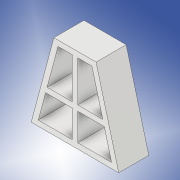
# Autodesk Inventor part: CA001
Saved by Autodesk Inventor 2017 (Build 210142000, 142)
## iProperties
Created: 2017-06-04
Part Number: CA001
Material: ABS Plastic
Document SubType Name: Modeling
Designer: Zach
Density: 1.06 g/cm^3
Appearance: CR White
Author: Zach
Autodesk Inventor part; units mm, degrees
ref_plane "YZ Plane" through (0, 0, 0) normal (1, 0, 0) x (0, 1, 0)
ref_plane "XZ Plane" through (0, 0, 0) normal (0, 1, 0) x (-1, 0, 0)
ref_plane "XY Plane" through (0, 0, 0) normal (0, 0, 1) x (1, 0, 0)
sketch "Sketch1" plane through (0, 0, 0) normal (0, 0, 1) x (1, 0, 0)
  line L0 (0, 0) -> (160, 0)
  line L1 (160, 0) -> (118.589, 154.5481)
  line L2 (41.411, 154.5481) -> (0, 0)
  line L3 (41.411, 154.5481) -> (118.589, 154.5481)
  dimension "d0" = 160
  dimension "d1" = 160
  dimension "d2" = 75
  dimension "d8" = 75
  constraints: 8 end point, 2 horizontal
  measures "d0" distance of L0.start L0.end
  measures "d1" distance of L1.end L0.end
  measures "d2" angle of L1 L0
  measures "d8" angle of L0 L2
extrude "Extrusion1" add sketch "Sketch1" along normal blind 55
sketch "Sketch6" plane through (0, 0, 55) normal (0, 0, 1) x (1, 0, 0)
  line L0 (0, 0) -> (160, 0) construction
  line L1 (160, 0) -> (118.589, 154.5481) construction
  line L2 (118.589, 154.5481) -> (41.411, 154.5481) construction
  line L3 (41.411, 154.5481) -> (0, 0) construction
  line L4 (110.9157, 144.5481) -> (146.9677, 10) construction
  line L5 (146.9677, 10) -> (13.0323, 10) construction
  line L6 (13.0323, 10) -> (49.0843, 144.5481) construction
  line L7 (49.0843, 144.5481) -> (110.9157, 144.5481) construction
  line L8 (85, 144.5481) -> (75, 144.5481) construction
  line L9 (75, 144.5481) -> (75, 10) construction
  line L10 (75, 10) -> (85, 10) construction
  line L11 (85, 10) -> (85, 144.5481) construction
  line L12 (133.5703, 60) -> (26.4297, 60) construction
  line L13 (26.4297, 60) -> (26.4297, 70) construction
  line L14 (26.4297, 70) -> (133.5703, 70) construction
  line L15 (133.5703, 70) -> (133.5703, 60) construction
  line L16 (133.5703, 60) -> (146.9677, 10)
  line L17 (85, 10) -> (146.9677, 10)
  line L18 (0, 0) -> (160, 0) construction
  line L19 (133.5703, 60) -> (85, 60)
  line L20 (85, 60) -> (85, 10)
  line L21 (75, 10) -> (75, 60)
  line L22 (26.4297, 60) -> (75, 60)
  line L23 (26.4297, 60) -> (13.0323, 10)
  line L24 (13.0323, 10) -> (75, 10)
  line L25 (75, 70) -> (75, 144.5481)
  line L26 (75, 144.5481) -> (49.0843, 144.5481)
  line L27 (75, 70) -> (29.1092, 70)
  line L28 (29.1092, 70) -> (49.0843, 144.5481)
  line L29 (85, 144.5481) -> (110.9157, 144.5481)
  line L30 (110.9157, 144.5481) -> (130.8908, 70)
  line L31 (130.8908, 70) -> (85, 70)
  line L32 (85, 70) -> (85, 144.5481)
  point P0 (80, 10)
  dimension "d22" = 10
  dimension "d23" = 10
  dimension "d24" = 10
  dimension "d25" = 50
  constraints: 56 end point, 16 point on line, 6 collinear, 6 parallel, 3 perpendicular, 2 horizontal, 2 midpoint, 3 other
  measures "d22" distance between parallel lines of L1 L4
  measures "d23" distance between parallel lines of L9 L11
  measures "d24" distance of L12.end L13.end
  measures "d25" distance between parallel lines of L5 L12
extrude "Extrusion5" cut sketch "Sketch6" against normal through all
body "Solid1"
